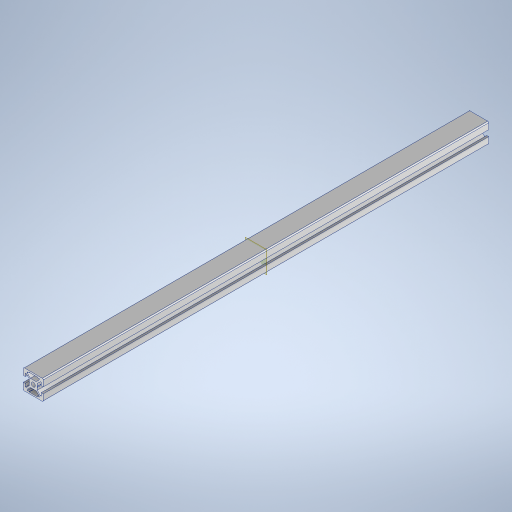
# Autodesk Inventor part: HFSH5-2020-446
Saved by Autodesk Inventor 2024 (Build 280153000, 153)
## iProperties
Category: PARTsolutions
Company: MISUMI
Created: 2024-12-26
Part Number: HFSH5-2020-446
Material: Aluminum 6061
Catalog Web Link: www.cadenas.de
Description: NFS5-2020, NFSB5-2020, HFS5-2020, HFSB5-2020, CAF5-2020, HFSY5-2020, NFSF5-2020, HFSF5-2020, HFSFB5-2020, NFST5-2020, HFST5-2020, HFSTB5-2020, HFSH5-2020, HFSC5-2020-HFS5 Series Aluminum Extrusions 20 Square -1 Slot-
Vendor: MISUMI
Document SubType Name: Modeling
Designer: psAdmin
Manufacturer: MISUMI
Mass: 260.401 g
Surface Area: 934.446 cm^2
Volume: 96.4447 cm^3
Density: 2.7 g/cm^3
Appearance: Aluminum - Flat
PSOL_IDENT_0: {$CADENAS_DATA/23d-libs/misumi/metric/38_al_extrusions_blackets/5/hfs5_2020.prj},679 {VTYP=3D},{NB=H
PSOL_IDENT_1: FSH5-2020-486},{LINA=HFSH5-2020-486},{NN=NFS5-2020, NFSB5-2020, HFS5-2020, HFSB5-2020, CAF5-2020, HF
PSOL_IDENT_2: SY5-2020, NFSF5-2020, HFSF5-2020, HFSFB5-2020, NFST5-2020, HFST5-2020, HFSTB5-2020, HFSH5-2020, HFSC
PSOL_IDENT_3: 5-2020},{DATE=08.05.2023 08:39:06},{GEOMDATE=27.07.2021 03:20:00},{VERSION=},{LINEID=170},{WBVAR=L,A
PSOL_IDENT_4: LT1,ALT2,ALT4,ALT5,CP5,DL5,DR5,ALT6,ALT9,ALT10,ALT11,HP6,NHL6,DL6,NHR6,DR6,ALT7,ALT8,NH9,AH,BH,CH,DH
PSOL_IDENT_5: ,EH,NH10,AV,BV,CV,DV,EV,NH11,AP,BP,CP,DP,EP,ALT12,ALT13,Z,NH12,XA,XB,XC,XD,XE,NH13,YA,YB,YC,YD,YE,AL
PSOL_IDENT_6: T16,HP16,DL16,DR16,ALT17,HQ17,JLP,ALT20},{WBNUMERIC=L,NH9,AH,BH,CH,DH,EH,NH10,AV,BV,CV,DV,EV,NH11,AP
PSOL_IDENT_7: ,BP,CP,DP,EP,NH12,XA,XB,XC,XD,XE,NH13,YA,YB,YC,YD,YE,HQ17,JLP}  {NB=HFSH5-2020-486},{LINA=HFSH5-2020
PSOL_IDENT_8: -486},{KT=DUMMY},{PN=HFSH5-2020-486},{TPS=HFSH5-2020},{MAT=A6N01SS-T5 Aluminum Alloy or 6005A-T5 Alu
PSOL_IDENT_9: minum Alloy},{ST=Clear Anodize},{FRMW=20},{FRMH=20},{FRD=4.2},{L=486},{MASS=0.53},{SA=199},{LX=0.74x
PSOL_IDENT_10: 10^4},{LY=0.89x10^4},{ALT1=},{M1=0},{DPL1=0},{DPR1=0},{ALT1PN=},{ALT2=},{ALT2ALG= '','w/o End Tappin
PSOL_IDENT_11: g (Heli-Coil Insert)','LHP','with LHP (Tapping on the Left (Heli-Coil Insert))','RHP','with RHP (Tap
PSOL_IDENT_12: ping on the Right (Heli-Coil Insert))','HPW','with HPW (Tapping on Both Ends (Heli-Coil Insert))' },
PSOL_IDENT_13: {M2=0},{DP2=0},{ALT2PN=},{ALT4=},{ALT4ALG= '', 'w/o SC (High Precision Cut)', 'SC', 'with SC (High P
PSOL_IDENT_14: recision Cut)' },{ALT4PN=},{ALT5=},{ALT5ALG= '','w/o 45 Degree Cut','1','with 45 Degree Cut' },{CP5=
PSOL_IDENT_15: },{CP5ALG= '','N/A' },{DL5=},{DL5ALG= '','N/A' },{DR5=},{DR5ALG= '','N/A' },{FRMLALT5=0},{FRMRALT5=0
PSOL_IDENT_16: },{ALT5PN=},{ALT6=},{ALT6ALG= '','w/o Fastening Location Wrench Access Hole Alterations','1','with F
PSOL_IDENT_17: astening Location Wrench Access Hole Alterations' },{ALT9=},{ALT9ALG= '','w/o Location Specified Wre
PSOL_IDENT_18: nch Access Hole Alteratons (Horizontal)','1','with Location Specified Wrench Access Hole Alteratons
PSOL_IDENT_19: (Horizontal)' },{ALT10=},{ALT10ALG= '','w/o Location Specified Wrench Access Hole Alteratons (Vertic
PSOL_IDENT_20: al)','1','with Location Specified Wrench Access Hole Alteratons (Vertical)' },{ALT11=},{ALT11ALG= ''
PSOL_IDENT_21: ,'w/o Location Specified Wrench Access Hole Alteratons (Crisscross)','1','with Location Specified Wr
PSOL_IDENT_22: ench Access Hole Alteratons (Crisscross)' },{HP6=},{HP6ALG= '','N/A' },{NHL6=},{NHL6ALG= '','N/A' },
PSOL_IDENT_23: {DL6=},{DL6ALG= '','N/A' },{NHR6=},{NHR6ALG= '','N/A' },{DR6=},{DR6ALG= '','N/A' },{HL6=0.000},{HL6D=
PSOL_IDENT_24: 0},{HR6=0.000},{HR6D=0},{J6=0},{J6D=0},{K6=0},{K6D=0},{DD6=0.00},{DD6ALG=0},{ALT7=},{ALT7ALG= '','N/
PSOL_IDENT_25: A' },{ALT8=},{ALT8ALG= '','N/A' },{ALT678PN=},{NH9=0},{NH9MAX=5},{NH9ALG=[0]},{AH=0.0},{AHMIN=7},{AH
PSOL_IDENT_26: MAX=481},{AHALG=[0]},{BH=0.0},{BHMIN=2},{BHMAX=483},{BHALG=[0]},{CH=0.0},{CHMIN=2},{CHMAX=485},{CHAL
PSOL_IDENT_27: G=[0]},{DH=0.0},{DHMIN=2},{DHMAX=487},{DHALG=[0]},{EH=0.0},{EHMIN=2},{EHMAX=479},{EHALG=[0]},{NH10=0
PSOL_IDENT_28: },{NH10MAX=5},{NH10ALG=[0]},{AV=0.0},{AVMIN=7},{AVMAX=481},{AVALG=[0]},{BV=0.0},{BVMIN=2},{BVMAX=483
PSOL_IDENT_29: },{BVALG=[0]},{CV=0.0},{CVMIN=2},{CVMAX=485},{CVALG=[0]},{DV=0.0},{DVMIN=2},{DVMAX=487},{DVALG=[0]},
PSOL_IDENT_30: {EV=0.0},{EVMIN=2},{EVMAX=479},{EVALG=[0]},{NH11=0},{NH11MAX=5},{NH11ALG=[0]},{AP=0.0},{APMIN=7},{AP
PSOL_IDENT_31: MAX=481},{APALG=[0]},{BP=0.0},{BPMIN=2},{BPMAX=483},{BPALG=[0]},{CP=0.0},{CPMIN=2},{CPMAX=485},{CPAL
PSOL_IDENT_32: G=[0]},{DP=0.0},{DPMIN=2},{DPMAX=487},{DPALG=[0]},{EP=0.0},{EPMIN=2},{EPMAX=479},{EPALG=[0]},{ALT9PN=
PSOL_IDENT_33: },{ALT10PN=},{ALT11PN=},{ALT91011PN=},{ALT12=},{ALT12ALG= '','N/A' },{ALT13=},{ALT13ALG= '','w/o Cou
PSOL_IDENT_34: nterbore Hole in Specified Position (Horizontal)','1','with Counterbore Hole in Specified Position (
PSOL_IDENT_35: Horizontal)' },{Z=},{ZALG= '','N/A' },{DD12=0.0},{DD112=0.0},{NH12=0},{NH12MAX=5},{NH12ALG=[0]},{XA=
PSOL_IDENT_36: 0.0},{XAMIN=7},{XAMAX=481},{XAALG=[0]},{XB=0.0},{XBMIN=2},{XBMAX=483},{XBALG=[0]},{XC=0.0},{XCMIN=2}
PSOL_IDENT_37: ,{XCMAX=485},{XCALG=[0]},{XD=0.0},{XDMIN=2},{XDMAX=487},{XDALG=[0]},{XE=0.0},{XEMIN=2},{XEMAX=479},{
PSOL_IDENT_38: XEALG=[0]},{NH13=0},{NH13MAX=5},{NH13ALG=[0]},{YA=0.0},{YAMIN=7},{YAMAX=481},{YAALG=[0]},{YB=0.0},{Y
PSOL_IDENT_39: BMIN=2},{YBMAX=483},{YBALG=[0]},{YC=0.0},{YCMIN=2},{YCMAX=485},{YCALG=[0]},{YD=0.0},{YDMIN=2},{YDMAX=
PSOL_IDENT_40: 487},{YDALG=[0]},{YE=0.0},{YEMIN=2},{YEMAX=479},{YEALG=[0]},{ALT12PN=},{ALT13PN=},{ALT1213PN=},{ALT1
PSOL_IDENT_41: 6=},{ALT16ALG= '','w/o M Type Hole Alteration','1','with M Type Hole Alteration' },{HP16=},{HP16ALG=
PSOL_IDENT_42: '','N/A' },{DL16=},{DL16ALG= '','N/A' },{DR16=},{DR16ALG= '','N/A' },{H116=0},{D16=0.0},{ALT16PN=},
PSOL_IDENT_43: {ALT17=},{ALT17ALG= '','N/A' },{HQ17=0},{HQ17ALG=0},{JLP=0},{JLPMIN=4.9},{JLPMAX=0},{JLPALG=[0]},{L1
PSOL_IDENT_44: 7=0},{D17=0.0},{ALT17PN=},{ALT20=},{ALT20PN=},{ERRORALT01=OK},{ERRORALT02=OK},{ERRORALT05=OK},{ERROR
PSOL_IDENT_45: ALT06091=OK},{ERRORALT06092=OK},{ERRORALT06093=OK},{ERRORALT06094=OK},{ERRORALT06101=OK},{ERRORALT06
PSOL_IDENT_46: 102=OK},{ERRORALT06103=OK},{ERRORALT06104=OK},{ERRORALT06111=OK},{ERRORALT06112=OK},{ERRORALT06113=O
PSOL_IDENT_47: K},{ERRORALT06114=OK},{ERRORALT06121=OK},{ERRORALT06122=OK},{ERRORALT06123=OK},{ERRORALT06124=OK},{E
PSOL_IDENT_48: RRORALT06131=OK},{ERRORALT06132=OK},{ERRORALT06133=OK},{ERRORALT06134=OK},{ERRORALT0616=OK},{ERRORAL
PSOL_IDENT_49: T06171=OK},{ERRORALT06172=OK},{ERRORALT06173=OK},{ERRORALT0911=OK},{ERRORALT0913=OK},{ERRORALT0916=O
PSOL_IDENT_50: K},{ERRORALT0917=OK},{ERRORALT1011=OK},{ERRORALT1012=OK},{ERRORALT1016=OK},{ERRORALT1017=OK},{ERRORA
PSOL_IDENT_51: LT1112=OK},{ERRORALT1113=OK},{ERRORALT1116=OK},{ERRORALT1117=OK},{ERRORALT1216=OK},{ERRORALT1217=OK}
PSOL_IDENT_52: ,{ERRORALT1316=OK},{ERRORALT1317=OK},{ERRORALT1617=OK},{ERRORPN=},{TFW=0}
NB: HFSH5-2020-486
NN: NFS5-2020, NFSB5-2020, HFS5-2020, HFSB5-2020, CAF5-2020, HFSY5-2020, NFSF5-2020, HFSF5-2020, HFSFB5-2020, NFST5-2020, HFST5-2020, HFSTB5-2020, HFSH5-2020, HFSC5-2020
NT: HFS5 Series Aluminum Extrusions 20 Square -1 Slot-
NBSYN: $PN.
LINA: HFSH5-2020-486
CATALOG: Misumi
PN: HFSH5-2020-486
TPS: HFSH5-2020
MAT: A6N01SS-T5 Aluminum Alloy or 6005A-T5 Aluminum Alloy
ST: Clear Anodize
L: 486
MASS: 0.53
SA: 199
LX: 0.74x10^4
LY: 0.89x10^4
ALT1: w/o End Tapping
M1: 0
DPL1: 0
DPR1: 0
ALT2: w/o End Tapping (Heli-Coil Insert)
M2: 0
DP2: 0
ALT4: w/o SC (High Precision Cut)
ALT5: w/o 45 Degree Cut
CP5: N/A
DL5: N/A
DR5: N/A
ALT6: w/o Fastening Location Wrench Access Hole Alterations
ALT9: w/o Location Specified Wrench Access Hole Alteratons (Horizontal)
ALT10: w/o Location Specified Wrench Access Hole Alteratons (Vertical)
ALT11: w/o Location Specified Wrench Access Hole Alteratons (Crisscross)
HP6: N/A
NHL6: N/A
DL6: N/A
NHR6: N/A
DR6: N/A
HL6D: 0
HR6D: 0
J6D: 0
K6D: 0
DD6: 0
ALT7: N/A
ALT8: N/A
NH9: 0
AH: 0
BH: 0
CH: 0
DH: 0
EH: 0
NH10: 0
AV: 0
BV: 0
CV: 0
DV: 0
EV: 0
NH11: 0
AP: 0
BP: 0
CP: 0
DP: 0
EP: 0
ALT12: N/A
ALT13: w/o Counterbore Hole in Specified Position (Horizontal)
Z: N/A
DD12: 0
DD112: 0
NH12: 0
XA: 0
XB: 0
XC: 0
XD: 0
XE: 0
NH13: 0
YA: 0
YB: 0
YC: 0
YD: 0
YE: 0
ALT16: w/o M Type Hole Alteration
HP16: N/A
DL16: N/A
DR16: N/A
H116: 0
D16: 0
ALT17: N/A
HQ17: 0
JLP: 0
D17: 0
ALT20: w/o CW (End Face C Chamfering)
SUPPLIER: MISUMI
ARTICLENO: HFSH5-2020-486
BOMINFO: HFSH5-2020-486
CREATOR: CADENAS GmbH
Title: HFSH5-2020-486
Author: Cadenas PARTsolutions
Comments: HFS5 Series Aluminum Extrusions 20 Square -1 Slot-
Autodesk Inventor part; units mm, degrees
ref_plane "YZ Plane" through (0, 0, 0) normal (1, 0, 0) x (0, 1, 0)
ref_plane "XZ Plane" through (0, 0, 0) normal (0, 1, 0) x (-1, 0, 0)
ref_plane "XY Plane" through (0, 0, 0) normal (0, 0, 1) x (1, 0, 0)
sketch "Sketch_65" plane through (0, 0, 0) normal (0, 0, 1) x (1, 0, 0)
  arc A0 (-10, -9) -> (-9, -10) centre (-9, -9) ccw
  line L0 (-9, -10) -> (9, -10)
  arc A1 (9, -10) -> (10, -9) centre (9, -9) ccw
  line L1 (10, -9) -> (10, -3)
  line L2 (10, -3) -> (8, -3)
  line L3 (8, -3) -> (8, -6)
  line L4 (8, -6) -> (7.0607, -6)
  line L5 (7.0607, -6) -> (4, -2.9393)
  line L6 (4, -2.9393) -> (4, -0.5196)
  line L7 (4, -0.5196) -> (3.7, 0)
  line L8 (3.7, 0) -> (4, 0.5196)
  line L9 (4, 0.5196) -> (4, 2.9393)
  line L10 (4, 2.9393) -> (7.0607, 6)
  line L11 (7.0607, 6) -> (8, 6)
  line L12 (8, 6) -> (8, 3)
  line L13 (8, 3) -> (10, 3)
  line L14 (10, 3) -> (10, 9)
  arc A2 (10, 9) -> (9, 10) centre (9, 9) ccw
  line L15 (9, 10) -> (-9, 10)
  arc A3 (-9, 10) -> (-10, 9) centre (-9, 9) ccw
  line L16 (-10, 9) -> (-10, 3)
  line L17 (-10, 3) -> (-8, 3)
  line L18 (-8, 3) -> (-8, 6)
  line L19 (-8, 6) -> (-7.0607, 6)
  line L20 (-7.0607, 6) -> (-4, 2.9393)
  line L21 (-4, 2.9393) -> (-4, 0.5196)
  line L22 (-4, 0.5196) -> (-3.7, 0)
  line L23 (-3.7, 0) -> (-4, -0.5196)
  line L24 (-4, -0.5196) -> (-4, -2.9393)
  line L25 (-4, -2.9393) -> (-7.0607, -6)
  line L26 (-7.0607, -6) -> (-8, -6)
  line L27 (-8, -6) -> (-8, -3)
  line L28 (-8, -3) -> (-10, -3)
  line L29 (-10, -3) -> (-10, -9)
  line L30 (-6, 7.0607) -> (-2.9393, 4)
  line L31 (-2.9393, 4) -> (2.9393, 4)
  line L32 (2.9393, 4) -> (6, 7.0607)
  line L33 (6, 7.0607) -> (6, 8)
  line L34 (6, 8) -> (4, 8)
  line L35 (4, 8) -> (4, 8.5)
  line L36 (4, 8.5) -> (-4, 8.5)
  line L37 (-4, 8.5) -> (-4, 8)
  line L38 (-4, 8) -> (-6, 8)
  line L39 (-6, 8) -> (-6, 7.0607)
  line L40 (-6, -7.0607) -> (-6, -8)
  line L41 (-6, -8) -> (-4, -8)
  line L42 (-4, -8) -> (-4, -8.5)
  line L43 (-4, -8.5) -> (4, -8.5)
  line L44 (4, -8.5) -> (4, -8)
  line L45 (4, -8) -> (6, -8)
  line L46 (6, -8) -> (6, -7.0607)
  line L47 (6, -7.0607) -> (2.9393, -4)
  line L48 (2.9393, -4) -> (-2.9393, -4)
  line L49 (-2.9393, -4) -> (-6, -7.0607)
  constraints: 100 end point, 8 point on circle, 4 centre point
extrude "Extrusion1" add sketch "Sketch_65" against normal blind 446
sketch "Sketch2" plane through (0, 0, -446) normal (0, 0, -1) x (-1, 0, 0)
  point P0 (0, 0)
hole "Hole1" at (0, 0, -446) direction (0, 0, 1) diameter 4.2 depth 486
ref_plane "C1_XY" through (0, 0, 0) normal (0, 0, 1) x (1, 0, 0)
ref_plane "C1_YZ" through (0, 0, 0) normal (1, 0, 0) x (0, 1, 0)
ref_plane "C1_ZX" through (0, 0, 0) normal (0, 1, 0) x (0, 0, 1)
thread "Thread1" size "M5x0.8" class "6H" standard "ANSI Metric M Profile" length 10
thread "Thread2" size "M5x0.8" class "6H" standard "ANSI Metric M Profile" length 10
ref_plane "Work Plane4" through (0, 0, -223) normal (0, 0, -1) x (-1, 0, 0)
body "Solid1"
